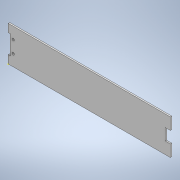
# Autodesk Inventor part: 220310 Back Cover
Saved by Autodesk Inventor 2022 (Build 260153000, 153)
## iProperties
Created: 2022-03-10
Part Number: 220310 Back Cover
Material: Generic
Document SubType Name: Modeling
Designer: josephinew
Density: 1 g/cm^3
Appearance: Default
Author: josephinew
Autodesk Inventor part; units mm, degrees
ref_plane "YZ Plane" through (0, 0, 0) normal (1, 0, 0) x (0, 1, 0)
ref_plane "XZ Plane" through (0, 0, 0) normal (0, 1, 0) x (-1, 0, 0)
ref_plane "XY Plane" through (0, 0, 0) normal (0, 0, 1) x (1, 0, 0)
sketch "Sketch1" plane through (0, 0, 0) normal (0, 0, 1) x (1, 0, 0)
  line L0 (0, 0) -> (352.552, 0)
  line L1 (352.552, 0) -> (352.552, 76.2)
  line L2 (352.552, 76.2) -> (0, 76.2)
  line L3 (0, 76.2) -> (0, 0)
  circle A0 centre (10.795, 51.308) radius 2.54
  circle A1 centre (10.795, 24.892) radius 2.54
  line L4 (102.1122, 0) -> (121.213, 0)
  line L5 (102.1122, 0) -> (83.0114, 0)
  line L6 (0, 76.2) -> (10.795, 76.2)
  line L7 (0, 63.0428) -> (0, 24.8412)
  line L8 (0, 76.2) -> (10.795, 76.2)
  line L9 (3.81, 38.1) -> (3.81, 58.1025)
  line L10 (3.81, 58.1025) -> (0, 58.1025)
  line L11 (3.81, 38.1) -> (3.81, 18.0975)
  line L12 (3.81, 18.0975) -> (0, 18.0975)
  line L13 (3.81, 38.1) -> (3.81, 58.1025)
  line L14 (0, 58.1025) -> (3.81, 58.1025)
  line L15 (3.81, 58.1025) -> (3.81, 18.0975)
  line L16 (3.81, 18.0975) -> (0, 18.0975)
  line L17 (0, 18.0975) -> (0, 58.1025)
  dimension "d0" = 352.552
  dimension "d1" = 76.2
  dimension "d15" = 20.0025
  constraints: 36 end point, 4 parallel, 4 perpendicular, 3 horizontal, 3 point on line, 2 centre point, 2 collinear, 2 vertical
  measures "d0" distance of L2.end L1.end
  measures "d1" distance of L1.end L0.end
  measures "d15" distance of L9.start L9.end
extrude "Extrusion1" add sketch "Sketch1" along normal blind 3.175
sketch "Sketch2" plane through (0, 0, 3.175) normal (0, 0, 1) x (1, 0, 0)
  line L0 (352.552, 76.2) -> (0, 76.2) projected
  line L1 (352.552, 0) -> (352.552, 76.2) projected
  line L2 (352.552, 50.8) -> (339.852, 50.8)
  line L3 (339.852, 50.8) -> (339.852, 25.4)
  line L4 (339.852, 25.4) -> (352.552, 25.4)
  line L5 (352.552, 25.4) -> (352.552, 50.8)
  point P0 (0, 0)
  dimension "d6" = 25.4
  dimension "d7" = 12.7
  dimension "d8" = 25.4
  constraints: 8 end point, 2 parallel, 1 horizontal, 1 perpendicular, 1 point on line
  measures "d6" distance of L0.start L2.start
  measures "d7" distance of L4.end L3.end
  measures "d8" distance of L3.end L2.end
extrude "Extrusion2" cut sketch "Sketch2" against normal blind 25.4
sketch "Sketch3" plane through (0, 0, 3.175) normal (0, 0, 1) x (1, 0, 0)
  point P0 (0, 0)
sketch "Sketch4" plane through (0, 0, 3.175) normal (0, 0, 1) x (1, 0, 0)
  point P0 (0, 0)
sketch "Sketch5" plane through (0, 0, 3.175) normal (0, 0, 1) x (1, 0, 0)
  circle A0 centre (10.795, 51.308) radius 2.54 projected
  circle A1 centre (10.795, 24.892) radius 2.54 projected
  line L0 (0, 76.2) -> (0, 0) projected
  line L1 (0, 38.1) -> (0, 58.7375)
  line L2 (0, 58.7375) -> (4.3688, 58.7375)
  line L3 (4.3688, 58.7375) -> (4.3688, 17.4625)
  line L4 (4.3688, 17.4625) -> (0, 17.4625)
  line L5 (0, 17.4625) -> (0, 38.1)
  point P0 (0, 17.4625)
  dimension "d16" = 20.6375
  dimension "d17" = 4.3688
  constraints: 10 end point, 4 perpendicular, 1 midpoint, 1 point on line
  measures "d16" distance of L1.start L1.end
  measures "d17" distance of L1.end L2.end
extrude "Extrusion3" cut sketch "Sketch5" against normal blind 25.4 contours L2 L3 L4 L0
sketch "Sketch6" plane through (0, 0, 3.175) normal (0, 0, 1) x (1, 0, 0)
  line L0 (352.552, 50.8) -> (352.552, 76.2) projected
  line L1 (0, 0) -> (352.552, 0) projected
  line L2 (352.552, 76.2) -> (350.647, 76.2)
  line L3 (350.647, 76.2) -> (350.647, 0)
  line L4 (350.647, 0) -> (352.552, 0)
  line L5 (352.552, 0) -> (352.552, 76.2)
  point P0 (352.552, 0)
  dimension "d21" = 1.905
  constraints: 8 end point, 2 parallel, 1 horizontal, 1 perpendicular, 1 point on line
  measures "d21" distance of L4.end L3.end
extrude "Extrusion4" cut sketch "Sketch6" against normal blind 25.4
body "Solid1"
